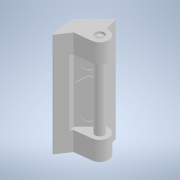
# Autodesk Inventor part: JB_HINGE
Saved by Autodesk Inventor 2021 (Build 250183000, 183)
## iProperties
Created: 2025-08-10
Part Number: JB_HINGE
Material: Generic
Catalog Web Link: www.cadenas.de
Description: JB HINGE-JB
Vendor: RITTAL
Document SubType Name: Modeling
Designer: psAdmin
Manufacturer: RITTAL
Mass: 2.48888 g
Surface Area: 18.6197 cm^2
Volume: 2.48888 cm^3
Density: 1 g/cm^3
Appearance: PSOLRGB-175-175-175
Category: PARTsolutions
Company: RITTAL
Title: JB_HINGE
Author: Cadenas PARTsolutions
Comments: JB
PSOL_IDENT_0: {$CADENAS_DATA/23d-libs/rittal/schaltschranksys/kleingeh/jb_parts/jb_hinge.prj},158 {VTYP=3D},{NB=JB
PSOL_IDENT_1: _HINGE},{LINA=JB_HINGE},{NN=JB HINGE},{DATE=20.08.2024 09:27:20},{GEOMDATE=03.07.2019 13:23:23},{VER
PSOL_IDENT_2: SION=},{LINEID=10},{WBVAR=},{WBNUMERIC=}  {NB=JB_HINGE},{LINA=JB_HINGE},{KT=DUMMY},{PN=JB_HINGE},{MT=
PSOL_IDENT_3: cs},{DETAIL=MIN}
NB: JB_HINGE
NN: JB HINGE
NT: JB
NBSYN: $PN.
LINA: JB_HINGE
CATALOG: Rittal
PN: JB_HINGE
MT: cs
DETAIL: 0
SUPPLIER: RITTAL
ARTICLENO: JB_HINGE
BOMINFO: JB_HINGE
CREATOR: CADENAS GmbH
Autodesk Inventor part; units mm, degrees
sketch "Sketch_1" plane through (0, 0, 0) normal (0, 1, 0) x (-1, 0, 0)
  line L0 (9.1622, -0.2102) -> (8.4597, 7.1326)
  line L1 (8.4597, 7.1326) -> (8.2577, 7.6457)
  arc A0 (8.2577, 7.6457) -> (7.905, 7.6831) centre (8.0716, 7.5725) ccw
  line L2 (7.905, 7.6831) -> (5.2627, 3.7047)
  arc A1 (5.1192, 3.6167) -> (5.2627, 3.7047) centre (5.0961, 3.8154) ccw
  line L3 (5.1192, 3.6167) -> (-0.3472, 2.9798)
  arc A2 (-0.3472, 2.9798) -> (0.287, -2.9862) centre (0, 0) ccw
  arc A3 (0.8188, -3.3585) -> (0.287, -2.9862) centre (0.3348, -3.4839) ccw
  line L4 (0.8188, -3.3585) -> (1.8215, -7.2275)
  arc A4 (1.8215, -7.2275) -> (2.1565, -7.3187) centre (2.0151, -7.1773) ccw
  line L5 (2.1565, -7.3187) -> (9.1045, -0.3707)
  arc A5 (9.1045, -0.3707) -> (9.1513, -0.2969) centre (8.9631, -0.2293) ccw
  arc A6 (9.1513, -0.2969) -> (9.1622, -0.2102) centre (8.9631, -0.2293) ccw
  circle A7 centre (0, 0) radius 1.555
  constraints: 14 point on circle, 12 end point, 8 centre point
extrude "Extrusion1" add sketch "Sketch_1" along normal mid plane 35
sketch "Sketch_2" plane through (0, 0, 0) normal (0, 1, 0) x (-1, 0, 0)
  line L0 (6.2296, 2.6092) -> (5.9185, 2.9204)
  line L1 (5.9185, 2.9204) -> (5.7646, 4.4605)
  line L2 (5.7646, 4.4605) -> (5.2627, 3.7047)
  line L3 (5.2627, 3.7047) -> (5.1192, 3.6167)
  line L4 (5.1192, 3.6167) -> (-0.3472, 2.9798)
  arc A0 (-0.3472, 2.9798) -> (0.287, -2.9862) centre (0, 0) ccw
  arc A1 (0.8188, -3.3585) -> (0.287, -2.9862) centre (0.3348, -3.4839) ccw
  line L5 (0.8188, -3.3585) -> (0.7763, -2.9407)
  arc A2 (0.9064, -2.714) -> (0.7763, -2.9407) centre (1.26, -3.0675) ccw
  line L6 (0.9064, -2.714) -> (6.2296, 2.6092)
  constraints: 14 end point, 6 point on circle, 3 centre point
extrude "Extrusion2" cut sketch "Sketch_2" along normal mid plane 22.1
sketch "Sketch_3" plane through (-0.9064, -11.05, -2.714) normal (0.7071, 0, 0.7071) x (-0.7071, 0, 0.7071)
  line L0 (0.334, -13.0303) -> (3.764, -15.0106)
  line L1 (3.764, -15.0106) -> (7.194, -13.0303)
  line L2 (7.194, -13.0303) -> (7.194, -9.0697)
  line L3 (7.194, -9.0697) -> (3.764, -7.0894)
  line L4 (3.764, -7.0894) -> (0.334, -9.0697)
  line L5 (0.334, -9.0697) -> (0.334, -13.0303)
  constraints: 12 end point
extrude "Extrusion3" add sketch "Sketch_3" along normal mid plane 0.6
sketch "Sketch_4" plane through (0, 0, 0) normal (1, 0, 0) x (0, 1, 0)
  line L0 (-17.5, 0) -> (17.5, 0)
  line L1 (17.5, 0) -> (17.5, -0.72)
  line L2 (17.5, -0.72) -> (16.75, -1.555)
  line L3 (16.75, -1.555) -> (-16.75, -1.555)
  line L4 (-16.75, -1.555) -> (-17.5, -0.72)
  line L5 (-17.5, -0.72) -> (-17.5, 0)
  line L6 (-17.5, 0) -> (17.5, 0)
  constraints: 14 end point
revolve "Revolution1" add sketch "Sketch_4" angle 360 about axis through (0, -17.5, 0) along (0, -1, 0)
sketch "Sketch5" plane through (-6.2296, -11.05, 2.6092) normal (0.7071, 0, 0.7071) x (0.7071, 0, -0.7071)
  point P0 (3.7632, 3.55)
hole "Hole1" at (-3.5687, -7.5, -0.0517) direction (-0.7071, 0, -0.7071) diameter 4.21 depth 0.2
sketch "Sketch6" plane through (-6.2296, -11.05, 2.6092) normal (0.7071, 0, 0.7071) x (0.7071, 0, -0.7071)
  point P0 (3.7632, 18.55)
hole "Hole2" at (-3.5687, 7.5, -0.0517) direction (-0.7071, 0, -0.7071) diameter 4.21 depth 0.2
ref_plane "to_bolt_XY" through (-3.5679, 0, -0.0524) normal (0.7071, 0, 0.7071) x (-0.7071, 0, 0.7071)
ref_plane "to_bolt_YZ" through (-3.5679, 0, -0.0524) normal (-0.7071, 0, 0.7071) x (0, -1, 0)
ref_plane "to_bolt_ZX" through (-3.5679, 0, -0.0524) normal (0, -1, 0) x (0.7071, 0, 0.7071)
ref_plane "to_door_XY" through (0, 0, 0) normal (0, 1, 0) x (1, 0, 0)
ref_plane "to_door_YZ" through (0, 0, 0) normal (1, 0, 0) x (0, 0, -1)
ref_plane "to_door_ZX" through (0, 0, 0) normal (0, 0, -1) x (0, 1, 0)
ref_plane "to_frame_XY" through (-5.6305, 0, -3.8447) normal (0.7071, 0, 0.7071) x (0.7071, 0, -0.7071)
ref_plane "to_frame_YZ" through (-5.6305, 0, -3.8447) normal (0.7071, 0, -0.7071) x (0, 1, 0)
ref_plane "to_frame_ZX" through (-5.6305, 0, -3.8447) normal (0, 1, 0) x (0.7071, 0, 0.7071)
body "Solid1"
